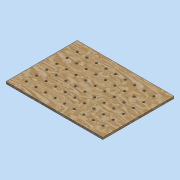
# Autodesk Inventor part: Sklejka stołu
Saved by Autodesk Inventor 2018 (Build 220112000, 112)
## iProperties
Created: 2019-01-25
Part Number: Sklejka stołu
Material: Ogólny
Document SubType Name: Modeling
Designer: Dawid
Density: 1 g/cm^3
Appearance: Sklejka — sezonowana
Author: Dawid
Autodesk Inventor part; units mm, degrees
ref_plane "YZ Plane" through (0, 0, 0) normal (1, 0, 0) x (0, 1, 0)
ref_plane "XZ Plane" through (0, 0, 0) normal (0, 1, 0) x (-1, 0, 0)
ref_plane "XY Plane" through (0, 0, 0) normal (0, 0, 1) x (1, 0, 0)
sketch "Szkic1" plane through (0, 0, 0) normal (0, 0, 1) x (1, 0, 0)
  line L0 (-475, -350) -> (475, -350)
  line L1 (475, -350) -> (475, 350)
  line L2 (475, 350) -> (-475, 350)
  line L3 (-475, 350) -> (-475, -350)
  line L4 (-475, -350) -> (475, 350) construction
  line L5 (475, -350) -> (-475, 350) construction
  point P0 (0, 0)
  dimension "d0" = 950
  dimension "d1" = 700
  constraints: 12 end point, 2 midpoint, 2 parallel, 1 horizontal, 1 perpendicular
  measures "d0" distance of L2.end L1.end
  measures "d1" distance of L1.end L0.end
extrude "Wyciągnięcie proste1" add sketch "Szkic1" along normal blind 20
sketch "Szkic2" plane through (0, 0, 20) normal (0, 0, 1) x (1, 0, 0)
  line L0 (-475, -350) -> (475, -350) projected
  line L1 (475, -350) -> (475, 350) projected
  line L2 (475, 350) -> (-475, 350) projected
  line L3 (-475, 350) -> (-475, -350) projected
  line L4 (-475, -350) -> (475, -350) projected
  line L5 (-475, -350) -> (-375, -350)
  line L6 (-475, -350) -> (-375, -350) construction
  line L7 (-375, -350) -> (-375, 350)
  line L8 (-375, -350) -> (-375, -250)
  circle A0 centre (-375, -250) radius 10
  point P0 (0, 0)
  dimension "d4" = 100
  dimension "d5" = 0
  dimension "d6" = 100
  dimension "d7" = 20
  constraints: 8 end point, 2 collinear, 2 point on line, 1 centre point, 1 coincident, 1 horizontal, 1 perpendicular
  measures "d4" distance of L0.start L5.end
  measures "d5" distance between parallel lines of L5 L6
  measures "d6" distance of L5.end L8.end
  measures "d7" diameter of A0
extrude "Wyciągnięcie proste2" cut sketch "Szkic2" against normal up to next contours A0 L7 | L7 A0
pattern_linear "Szyk prostokątny1" count 6 spacing 100 along (0, 1, 0) count 9 spacing 94 along (1, 0, 0) of "Wyciągnięcie proste2"
